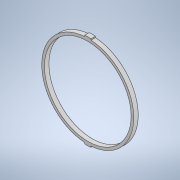
# Autodesk Inventor part: venti-valve-lock-ring
Saved by Autodesk Inventor 2020.2 (Build 242310000, 310)
## iProperties
Created: 2020-04-25
Part Number: venti-valve-lock-ring
Material: Generic
Document SubType Name: Modeling
Designer: iamin
Density: 1 g/cm^3
Appearance: Default
VLDS_Profile: Default Part
VLDS_TimeStamp: 2020-04-26
VLDS_FailCnt: 0
VLDS_AcceptCnt: 0
Author: iamin
Autodesk Inventor part; units mm, degrees
ref_plane "YZ Plane" through (0, 0, 0) normal (1, 0, 0) x (0, 1, 0)
ref_plane "XZ Plane" through (0, 0, 0) normal (0, 1, 0) x (-1, 0, 0)
ref_plane "XY Plane" through (0, 0, 0) normal (0, 0, 1) x (1, 0, 0)
sketch "Sketch1" plane through (0, 0, 0) normal (0, 0, 1) x (1, 0, 0)
  circle A0 centre (0, 0) radius 19.7
  line L0 (-1.435, 20.8507) -> (-1.435, 21.3507)
  line L1 (1.435, 21.3507) -> (1.435, 20.8507)
  arc A1 (1.435, 21.3507) -> (-1.435, 21.3507) centre (0, 12.6834) ccw
  line L2 (-5.669, 0) -> (4.2057, 0)
  line L3 (0, 24.0978) -> (0, 18.8809)
  line L4 (-1.435, -20.8507) -> (-1.435, -21.3507)
  line L5 (1.435, -21.3507) -> (1.435, -20.8507)
  arc A2 (-1.435, -21.3507) -> (1.435, -21.3507) centre (0, -12.6834) ccw
  arc A3 (-1.435, 20.8507) -> (-1.435, -20.8507) centre (0, 0) ccw
  arc A4 (1.435, -20.8507) -> (1.435, 20.8507) centre (0, 0) ccw
  dimension "d2" = 0.5
  dimension "d3" = 0.5
  dimension "d4" = 2.87
  constraints: 12 end point, 8 point on circle, 5 centre point, 5 symmetric about line, 2 vertical, 1 coincident, 1 horizontal, 1 point on line, 2 other
  measures "d2" distance of L0.start L0.end
  measures "d3" distance of L1.end L1.start
  measures "d4" distance of L1.start L0.end
extrude "Extrusion1" add sketch "Sketch1" along normal blind 2.03
body "Solid1"
